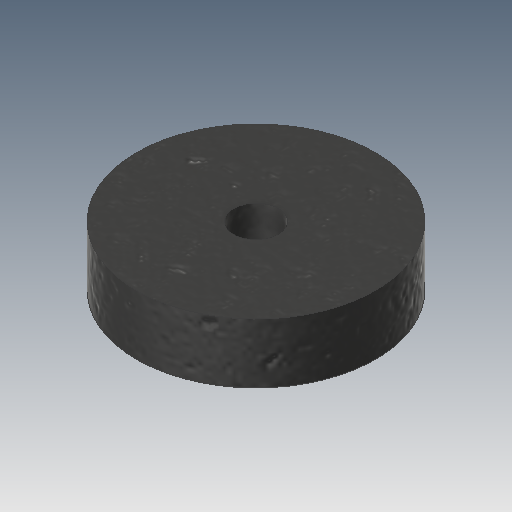
# Autodesk Inventor part: BASE VALVE
Saved by Autodesk Inventor 2019 (Build 230136000, 136)
## iProperties
Created: 2023-06-18
Part Number: BASE VALVE
Material: Generic
Document SubType Name: Modeling
Designer: Fransic
Density: 1 g/cm^3
Appearance: Fine Textured - Black
Mass: 28.1913 g
Surface Area: 68.7773 cm^2
Volume: 28.1913 cm^3
Author: Fransic
Autodesk Inventor part; units mm, degrees
ref_plane "YZ Plane" through (0, 0, 0) normal (1, 0, 0) x (0, 1, 0)
ref_plane "XZ Plane" through (0, 0, 0) normal (0, 1, 0) x (-1, 0, 0)
ref_plane "XY Plane" through (0, 0, 0) normal (0, 0, 1) x (1, 0, 0)
sketch "Sketch1" plane through (0, 0, 0) normal (0, 1, 0) x (-1, 0, 0)
  circle A0 centre (0, 0) radius 26.5
  dimension "d0" = 53
  constraints: 1 centre point, 1 coincident
  measures "d0" diameter of A0
extrude "Extrusion1" add sketch "Sketch1" along normal blind 13.25
sketch "Sketch2" plane through (0, 13.25, 0) normal (0, 1, 0) x (1, 0, 0)
  circle A0 centre (0, 0) radius 5
  dimension "d3" = 10
  constraints: 1 centre point, 1 coincident
  measures "d3" diameter of A0
extrude "Extrusion2" cut sketch "Sketch2" against normal through all
body "Solid1"
